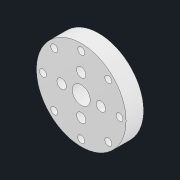
# Autodesk Inventor part: scara-base10
Saved by Autodesk Inventor 2022 (Build 260153000, 153)
## iProperties
Created: 2021-10-11
Part Number: scara-base10
Material: ABS プラスチック
Document SubType Name: Modeling
Designer: Yuta Kage
Density: 1.06 g/cm^3
Appearance: 滑らか - 白
Description: 印刷
Author: Yuta Kage
Autodesk Inventor part; units mm, degrees
ref_plane "YZ Plane" through (0, 0, 0) normal (1, 0, 0) x (0, 1, 0)
ref_plane "XZ Plane" through (0, 0, 0) normal (0, 1, 0) x (-1, 0, 0)
ref_plane "XY Plane" through (0, 0, 0) normal (0, 0, 1) x (1, 0, 0)
sketch "スケッチ1" plane through (0, 0, 0) normal (0, 0, 1) x (1, 0, 0)
  circle A0 centre (0, 0) radius 20.5
  dimension "d0" = 41
  constraints: 1 centre point, 1 coincident
  measures "d0" diameter of A0
extrude "押し出し1" add sketch "スケッチ1" along normal blind 8
sketch "スケッチ2" plane through (0, 0, 8) normal (0, 0, 1) x (1, 0, 0)
  circle A0 centre (0, 0) radius 17.5
  point P0 (0, 17.5)
  point P1 (-12.3744, 12.3744)
  point P2 (-17.5, 0)
  point P3 (-12.3744, -12.3744)
  point P4 (0, -17.5)
  point P5 (12.3744, -12.3744)
  point P6 (17.5, 0)
  point P7 (12.3744, 12.3744)
  dimension "d3" = 35
  dimension "d6" = 360
  constraints: 1 coincident, 1 vertical alignment, 11 other
hole "穴1" at (0, 17.5, 8) at (-12.3744, 12.3744, 8) at (-17.5, 0, 8) at (-12.3744, -12.3744, 8) at (0, -17.5, 8) at (12.3744, -12.3744, 8) at (17.5, 0, 8) at (12.3744, 12.3744, 8) direction (0, 0, -1) diameter 3.2 end through all clearance for "Socket Head Cap Screw" size "M3" standard "Ansi Metric M Profile"
sketch "スケッチ3" plane through (0, 0, 0) normal (0, 0, -1) x (-1, 0, 0)
  circle A0 centre (0, 0) radius 9
  point P0 (0, 9)
  point P1 (-9, 0)
  point P2 (0, -9)
  point P3 (9, 0)
  dimension "d15" = 18
  dimension "d18" = 360
  constraints: 1 coincident, 1 vertical alignment, 7 other
hole "穴2" at (0, 9, 0) at (9, 0, 0) at (0, -9, 0) at (-9, 0, 0) direction (0, 0, 1) diameter 4.3 end through all counterbore diameter 8 counterbore depth 4.2 clearance for "Socket Head Cap Screw" size "M4" standard "Ansi Metric M Profile"
sketch "スケッチ4" plane through (0, 0, 8) normal (0, 0, 1) x (1, 0, 0)
  circle A0 centre (0, 0) radius 4.1
  dimension "d27" = 8.2
  constraints: 1 centre point, 1 coincident
  measures "d27" diameter of A0
extrude "押し出し2" cut sketch "スケッチ4" against normal through all
